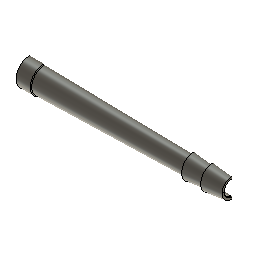
5mm-3mm Restrictor (Autodesk Fusion 360 design; units mm, degrees)
Autodesk Fusion 360 part; units mm, degrees
sketch "Sketch1" plane through (0, 0, 0) normal (0, 0, 1) x (1, 0, 0)
  line L0 (30, 0) -> (30, 3.6)
  line L1 (23, 0) -> (23, 4.5)
  line L2 (23, 4.5) -> (30, 3.6)
  line L3 (23, 0) -> (30, 0)
  dimension "d1" = 3.6
  dimension "d3" = 4.5
  constraint vertical L0
  constraint vertical L1
  constraint perpendicular L1 L3
  measures "d1" distance of L0.start L0.end
  measures "d3" distance of L1.start L1.end
revolve "Revolve1" add sketch "Sketch1" angle 360 about axis through (23, 0, 0) along (1, 0, 0) makes body 1
pattern_linear "R-Pattern1" count 2 spacing 7 along (-1, 0, 0) of bodies 1 makes body 2
ref_plane "WorkPlane1" through (-39, 0, 0) normal (-1, 0, 0) x (0, 0, 1)
sketch "Sketch3" plane through (16, 0, 0) normal (-1, 0, 0) x (0, -1, 0)
  circle A0 centre (0, 0) radius 4.5
  circle A1 centre (0, 0) radius 3.6
  dimension "d10" = 7.2
  constraint coincident A0.centre A1.centre
  measures "d10" diameter of A1
sketch "Sketch4" plane through (-39, 0, 0) normal (-1, 0, 0) x (0, -1, 0)
  circle A0 centre (0, 0) radius 1.5
  circle A1 centre (0, 0) radius 4.75
  dimension "d11" = 3
  dimension "d13" = 9.5
  constraint coincident A0.centre A1.centre
  constraint concentric A0 A1
  measures "d11" diameter of A0
  measures "d13" diameter of A1
sketch "Sketch5" plane through (30, 0, 0) normal (1, 0, 0) x (0, 1, 0)
  circle A0 centre (0, 0) radius 3.6
  circle A1 centre (0, 0) radius 2.6
  dimension "d12" = 5.2
  constraint concentric A0 A1
  measures "d12" diameter of A1
loft "Loft1" add profiles "Sketch3", "Sketch4" section 1 contours A1 section 2 contours A0 | A1 bodies 2
loft "Loft2" cut profiles "Sketch4", "Sketch5" section 1 contours A0 section 2 contours A1 bodies 1 2
sketch "Sketch6" plane through (-39, 0, 0) normal (-1, 0, 0) x (0, 0, 1)
  circle A0 centre (0, 0) radius 2.2254
  circle A1 centre (0, 0) radius 1.5
  arc A2 (1.42, 3.207) -> (-1.1139, 3.3257) centre (0, 0) ccw
  arc A3 (2.735, 2.9382) -> (1.42, 3.207) centre (1.417, -0.159) ccw
  arc A4 (-1.1139, 3.3257) -> (-2.6284, 3.1064) centre (-1.332, -0.506) ccw
  arc A5 (-1.42, -3.207) -> (1.1139, -3.3257) centre (0, 0) ccw
  arc A6 (-2.735, -2.9382) -> (-1.42, -3.207) centre (-1.417, 0.159) ccw
  arc A7 (1.1139, -3.3257) -> (2.6284, -3.1064) centre (1.332, 0.506) ccw
  line L0 (0, 0, 0) -> (0, 0, 5.5)
  circle A8 centre (0, 0) radius 4
  circle A9 centre (0, 0) radius 5
extrude "Extrude1" add sketch "Sketch6" along normal blind 7.5 draft -1.72 contours A0 | A1 bodies 2
extrude "Extrude2" cut sketch "Sketch6" along normal blind 7.5 contours A1 bodies 2
extrude "Extrude3" add sketch "Sketch6" along normal blind 5.5 contours A9 bodies 2
sweep "Sweep1" add twist angle 396 profiles "Sketch6" path "Sketch6" along L0 section 1 contours A2 A3 A4 A8 | A5 A6 A7 A8 bodies 2
chamfer "Chamfer1" distance 0.25 angle 45 1 edges at (-39, -1.8081, -4.6616) on bodies 2
combine "Combine1" operation add target body 1 tool bodies 2
chamfer "Chamfer2" distance 0.3 angle 45 1 edges at (30, -2.4241, 0.9402) on bodies 1
fillet "Fillet1" radius 0.4 1 edges at (29.7, 2.4196, -0.9385) on bodies 1
